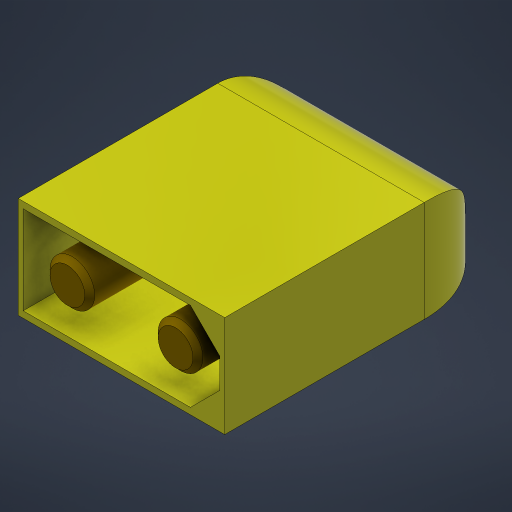
# Autodesk Inventor part: XT90PW
Saved by Autodesk Inventor 2023.5 (Build 275446000, 446)
## iProperties
Created: 2025-03-27
Part Number: XT90PW
Material: PC/ABS-Kunststoff
Document SubType Name: Modeling
Designer: David Lill
Density: 0.357273 g/cm^3
Appearance: Glatt - Gelb
Author: David Lill
Autodesk Inventor part; units mm, degrees
ref_plane "YZ Plane" through (0, 0, 0) normal (1, 0, 0) x (0, 1, 0)
ref_plane "XZ Plane" through (0, 0, 0) normal (0, 1, 0) x (-1, 0, 0)
ref_plane "XY Plane" through (0, 0, 0) normal (0, 0, 1) x (1, 0, 0)
sketch "Skizze1" plane through (0, 0, 0) normal (0, 0, 1) x (1, 0, 0)
  line L0 (0, 0) -> (20.8, 0)
  line L1 (20.8, 0) -> (20.8, 20.1)
  line L2 (20.8, 20.1) -> (0, 20.1)
  line L3 (0, 20.1) -> (0, 0)
  arc A0 (2.8586, 27.1) -> (0, 20.1) centre (10, 20.1) ccw
  line L4 (2.8586, 27.1) -> (17.9414, 27.1)
  arc A1 (20.8, 20.1) -> (17.9414, 27.1) centre (10.8, 20.1) ccw
  circle A2 centre (4.95, 24.4) radius 1.95
  circle A3 centre (15.85, 24.4) radius 1.95
  line L5 (4.95, 26.35) -> (15.85, 26.35) construction
  point P0 (10.4, 27.1)
  dimension "d4" = 3.9
  dimension "d0" = 27.1
  dimension "d1" = 20.8
  dimension "d2" = 7
  dimension "d3" = 10
  dimension "d5" = 10.9
  dimension "d6" = 5.45
  dimension "d7" = 26.35
  constraints: 12 end point, 4 horizontal, 4 point on circle, 2 centre point, 2 parallel, 2 tangent, 2 vertical alignment, 1 equal radius, 1 midpoint, 1 perpendicular, 4 other
  measures "d0" distance between parallel lines of L0 L4
  measures "d1" distance between parallel lines of L3 L1
  measures "d2" distance between parallel lines of L4 L2
  measures "d3" radius of A1
  measures "d5" distance of point (4.95, 24.4) point (15.85, 24.4)
  measures "d6" horizontal distance of point (10.4, 27.1) point (4.95, 24.4)
  measures "d7" distance between parallel lines of L0 L5
extrude "Extrusion1" add sketch "Skizze1" along normal blind 10.2 contours L3 L2 L1 L0 | A0 L4 A1 L2 | A2 | A3
extrude "Extrusion2" add sketch "Skizze1" against normal blind 3 contours A2 | A3
fillet "Rundung1" radius 7 1 edges at (10.4, 27.1, 10.2)
chamfer "Fase1" distance 0.5 angle 45 2 edges at (13.9, 24.4, -3) (3, 24.4, -3)
sketch "Skizze2" plane through (0, 0, 0) normal (0, -1, 0) x (1, 0, 0)
  line L0 (0.5, 0.65) -> (0.5, 9.55)
  line L1 (0.5, 9.55) -> (17.35, 9.55)
  line L2 (17.35, 9.55) -> (20.3, 6.6)
  line L3 (20.3, 6.6) -> (20.3, 3.6)
  line L4 (20.3, 3.6) -> (17.35, 0.65)
  line L5 (0.5, 0.65) -> (17.35, 0.65)
  line L6 (0, 0) -> (0, 10.2) projected
  circle A0 centre (4.95, 5.1) radius 2.85
  circle A1 centre (4.95, 5.1) radius 2.25
  circle A2 centre (15.85, 5.1) radius 2.85
  circle A3 centre (15.85, 5.1) radius 2.25
  line L7 (0, 10.2) -> (20.8, 10.2) projected
  point P0 (0.5, 5.1)
  point P1 (0, 5.1)
  point P2 (20.3, 5.1)
  point P3 (10.4, 10.2)
  dimension "d16" = 19.8
  dimension "d17" = 8.9
  dimension "d18" = 0.5
  dimension "d19" = 3
  dimension "d20" = 45
  dimension "d21" = 5.7
  dimension "d22" = 4.5
  dimension "d23" = 10.9
  dimension "d24" = 5.45
  constraints: 12 end point, 4 centre point, 4 horizontal alignment, 4 midpoint, 2 coincident, 2 equal radius, 2 perpendicular, 2 vertical, 1 horizontal, 1 vertical alignment
  measures "d16" distance between parallel lines of L0 L3
  measures "d17" distance between parallel lines of L5 L1
  measures "d18" distance between parallel lines of L6 L0
  measures "d19" distance of L2.end L3.end
  measures "d20" angle of L1 L2
  measures "d21" diameter of A0
  measures "d22" diameter of A1
  measures "d23" distance of A2.centre A0.centre
  measures "d24" horizontal distance of point (10.4, 10.2) A0.centre
extrude "Extrusion3" cut sketch "Skizze2" against normal blind 11 contours L0 L1 L2 L3 L4 L5 | A0 | A2
chamfer "Fase2" distance 0.5 angle 45 2 edges at (2.7, 0, 5.1) (13.6, 0, 5.1)
equation "\"d6\" = 0.5 * d5"
equation "\"d24\" = 0.5 * d23"
